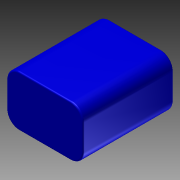
# Autodesk Inventor part: 276-1456
Saved by Autodesk Inventor 2013 (Build 170138000, 138)
## iProperties
Category: Power
Company: Autodesk Inc.
Created: 2012-02-01
Part Number: 276-1456
Document SubType Name: Modeling
Designer: Autodesk Inc.
Density: 1 g/cm^3
Catalog Web Link: http://www.vexrobotics.com/products/accessories/power/276-1456.html
Vendor: VEX
Material: Generic
Author: Autodesk Inc.
Autodesk Inventor part; units mm, degrees
ref_plane "YZ Plane" through (0, 0, 0) normal (1, 0, 0) x (0, 1, 0)
ref_plane "XZ Plane" through (0, 0, 0) normal (0, 1, 0) x (-1, 0, 0)
ref_plane "XY Plane" through (0, 0, 0) normal (0, 0, 1) x (1, 0, 0)
sketch "Sketch1" plane through (0, 0, 0) normal (0, 0, 1) x (1, 0, 0)
  line L0 (0, 0) -> (42.8752, 0)
  line L1 (42.8752, 0) -> (42.8752, 28.575)
  line L2 (42.8752, 28.575) -> (0, 28.575)
  line L3 (0, 28.575) -> (0, 0)
  dimension "d0" = 42.8752
  dimension "d1" = 28.575
  constraints: 8 end point, 2 parallel, 1 horizontal, 1 perpendicular
  measures "d0" distance of L2.end L1.end
  measures "d1" distance of L0.end L1.end
extrude "Extrusion1" add sketch "Sketch1" against normal blind 50.8
fillet "Fillet1" radius 7.1374 4 edges at (42.8752, 28.575, -25.4) (0, 28.575, -25.4) (0, 0, -25.4) (42.8752, 0, -25.4)
fillet "Fillet2" radius 0.8128 16 edges at (21.4376, 28.575, 0) (2.0905, 26.4845, 0) (0, 14.2875, 0) (2.0905, 2.0905, 0) (21.4376, 0, 0) (40.7847, 2.0905, 0) (42.8752, 14.2875, 0) (40.7847, 26.4845, 0) (21.4376, 28.575, -50.8) (2.0905, 26.4845, -50.8) (0, 14.2875, -50.8) (2.0905, 2.0905, -50.8) (21.4376, 0, -50.8) (40.7847, 2.0905, -50.8) (42.8752, 14.2875, -50.8) (40.7847, 26.4845, -50.8)
body "Solid1"
